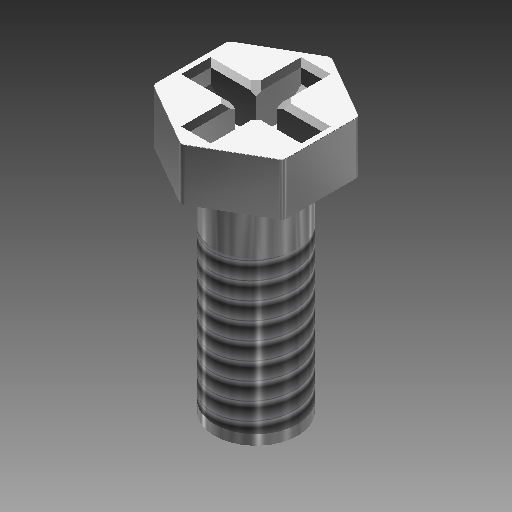
# Autodesk Inventor part: SSR-40 DA Screw
Saved by Autodesk Inventor 2019 (Build 230136000, 136)
## iProperties
Created: 2014-10-30
Part Number: SSR-40 DA Screw
Material: Nickel-Copper Alloy 400
Document SubType Name: Modeling
Designer: Tyler
Density: 8.83 g/cm^3
Appearance: Chrome - Polished
Mass: 1.52219 g
Surface Area: 2.59012 cm^2
Volume: 0.172388 cm^3
Author: Tyler
Autodesk Inventor part; units mm, degrees
ref_plane "YZ Plane" through (0, 0, 0) normal (1, 0, 0) x (0, 1, 0)
ref_plane "XZ Plane" through (0, 0, 0) normal (0, 1, 0) x (-1, 0, 0)
ref_plane "XY Plane" through (0, 0, 0) normal (0, 0, 1) x (1, 0, 0)
sketch "Sketch1" plane through (0, 0, 0) normal (0, 1, 0) x (-1, 0, 0)
  circle A0 centre (0, 0) radius 1.905
  dimension "d0" = 3.81
  constraints: 1 centre point, 1 coincident
  measures "d0" diameter of A0
extrude "Extrusion1" add sketch "Sketch1" along normal blind 9.9314
thread "Thread1" size "8-32 UNC" class "2A" standard "ANSI Unified Screw Threads" length 6.9342 offset 2.54
sketch "Sketch2" plane through (0, 9.9314, 0) normal (0, 1, 0) x (1, 0, 0)
  line L0 (0, -3.4544) -> (-2.9916, -1.7272)
  line L1 (-2.9916, -1.7272) -> (-2.9916, 1.7272)
  line L2 (-2.9916, 1.7272) -> (0, 3.4544)
  line L3 (0, 3.4544) -> (2.9916, 1.7272)
  line L4 (2.9916, 1.7272) -> (2.9916, -1.7272)
  line L5 (2.9916, -1.7272) -> (0, -3.4544)
  point P0 (0, 0)
  point P1 (0, 0)
  dimension "d7" = 6.9088
  constraints: 12 end point, 1 coincident, 13 other
  measures "d7" distance of L2.end L0.start
extrude "Extrusion2" add sketch "Sketch2" along normal blind 2.3876
fillet "Fillet1" radius 0.254 6 edges at (2.9916, 11.1252, -1.7272) (0, 11.1252, -3.4544) (-2.9916, 11.1252, -1.7272) (-2.9916, 11.1252, 1.7272) (2.9916, 11.1252, 1.7272) (0, 11.1252, 3.4544)
fillet "Fillet2" radius 0.0254 12 edges at (-2.9576, 12.319, 1.7076) (-1.4958, 12.319, 2.5908) (0, 12.319, 3.4151) (1.4958, 12.319, 2.5908) (2.9576, 12.319, 1.7076) (2.9916, 12.319, 0) (2.9576, 12.319, -1.7076) (1.4958, 12.319, -2.5908) (0, 12.319, -3.4151) (-1.4958, 12.319, -2.5908) (-2.9576, 12.319, -1.7076) (-2.9916, 12.319, 0)
sketch "Sketch3" plane through (0, 12.319, 0) normal (0, 1, 0) x (1, 0, 0)
  line L0 (2.54, 0.4699) -> (-2.54, 0.4699)
  line L1 (-2.54, 0.4699) -> (-2.54, -0.4699)
  line L2 (-2.54, -0.4699) -> (2.54, -0.4699)
  line L3 (2.54, -0.4699) -> (2.54, 0.4699)
  line L4 (0.4699, 2.54) -> (-0.4699, 2.54)
  line L5 (-0.4699, 2.54) -> (-0.4699, -2.54)
  line L6 (-0.4699, -2.54) -> (0.4699, -2.54)
  line L7 (0.4699, -2.54) -> (0.4699, 2.54)
  line L8 (2.9916, -1.5806) -> (2.9916, 1.5806) projected
  line L9 (-2.9662, -1.5806) -> (-2.9662, 1.5806) projected
  point P0 (0, 0)
  point P1 (2.54, 0)
  point P2 (-0.4699, 0)
  point P3 (0, -2.54)
  point P4 (0, -0.4699)
  dimension "d12" = 0.9398
  dimension "d13" = 0.9398
  dimension "d14" = 5.08
  dimension "d15" = 5.08
  dimension "d16" = 0.4516
  dimension "d17" = 0.4262
  constraints: 16 end point, 4 midpoint, 4 parallel, 2 horizontal, 2 horizontal alignment, 2 perpendicular, 2 vertical alignment
  measures "d12" distance of L2.end L0.start
  measures "d13" distance of L5.end L6.end
  measures "d14" distance of L6.end L4.start
  measures "d15" distance of L1.end L2.end
  measures "d16" distance between parallel lines of L8 L3
  measures "d17" distance between parallel lines of L9 L1
extrude "Extrusion3" cut sketch "Sketch3" against normal blind 1.8796
chamfer "Chamfer1" distance 0.2032 angle 45 12 edges at (-1.505, 12.319, -0.4699) (-1.505, 12.319, 0.4699) (-2.54, 12.319, 0) (-0.4699, 12.319, -1.505) (0, 12.319, -2.54) (0.4699, 12.319, -1.505) (1.505, 12.319, -0.4699) (2.54, 12.319, 0) (1.505, 12.319, 0.4699) (0.4699, 12.319, 1.505) (0, 12.319, 2.54) (-0.4699, 12.319, 1.505)
chamfer "Chamfer2" distance 0.2032 angle 45 4 edges at (-0.5715, 12.2174, -0.5715) (0.5715, 12.2174, -0.5715) (-0.5715, 12.2174, 0.5715) (0.5715, 12.2174, 0.5715)
chamfer "Chamfer3" distance 1.016 angle 45 1 edges at (2.54, 10.4394, 0)
chamfer "Chamfer4" distance 1.016 angle 45 3 edges at (0, 10.4394, 2.54) (-2.54, 10.4394, 0) (0, 10.4394, -2.54)
body "Solid1"
